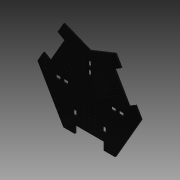
# Autodesk Inventor part: Bottom Plate
Saved by Autodesk Inventor 2015 (Build 190159000, 159)
## iProperties
Created: 2016-02-25
Part Number: Bottom Plate
Material: Polycarbonate, Clear
Document SubType Name: Modeling
Designer: James Yelland
Density: 1.2 g/cm^3
Appearance: Polycarbonate - Clear
Mass: 78.7459 g
Surface Area: 479.492 cm^2
Volume: 65.6216 cm^3
Author: James Yelland
Autodesk Inventor part; units mm, degrees
ref_plane "YZ Plane" through (0, 0, 0) normal (1, 0, 0) x (0, 1, 0)
ref_plane "XZ Plane" through (0, 0, 0) normal (0, 1, 0) x (-1, 0, 0)
ref_plane "XY Plane" through (0, 0, 0) normal (0, 0, 1) x (1, 0, 0)
sketch "Sketch1" plane through (0, 0, 0) normal (0, 1, 0) x (-1, 0, 0)
  line L0 (60.9555, 0.8544) -> (49.9555, 19.907)
  line L1 (-50.0445, 19.907) -> (-61.0445, 0.8544)
  line L2 (-28.0445, -153.2981) -> (-50.0445, -153.2981)
  line L3 (-50.0445, -153.2981) -> (-100.0445, -66.6956)
  line L4 (27.9555, -153.2981) -> (49.9555, -153.2981)
  line L5 (49.9555, -153.2981) -> (99.9555, -66.6956)
  line L6 (-100.0445, -66.6956) -> (-89.0445, -47.643)
  line L7 (88.9555, -47.643) -> (99.9555, -66.6956)
  line L8 (-0.0445, -0.093) -> (-50.0445, 19.907)
  line L9 (-0.0445, -0.093) -> (49.9555, 19.907)
  circle A0 centre (-66.9644, -113.992) radius 1.6
  circle A1 centre (-59.4644, -126.9824) radius 1.6
  circle A2 centre (59.3754, -126.9824) radius 1.6
  circle A3 centre (66.8754, -113.992) radius 1.6
  circle A4 centre (-49.2144, 11.3448) radius 1.6
  circle A5 centre (49.1254, 11.3448) radius 1.6
  circle A6 centre (-85.1445, -61.6956) radius 1.6
  circle A7 centre (-85.1445, -71.6956) radius 1.6
  circle A8 centre (85.0555, -61.6956) radius 1.6
  circle A9 centre (85.0555, -71.6956) radius 1.6
  circle A10 centre (-56.5116, -34.0943) radius 1.65
  circle A11 centre (-51.0123, -37.2693) radius 1.65
  circle A12 centre (-45.513, -40.4443) radius 1.65
  circle A13 centre (-40.0138, -43.6193) radius 1.65
  circle A14 centre (-34.5145, -46.7943) radius 1.65
  circle A15 centre (-29.0152, -49.9693) radius 1.65
  circle A16 centre (-23.516, -53.1443) radius 1.65
  circle A17 centre (-20.9056, -42.1229) radius 1.7
  circle A18 centre (-26.4048, -38.9479) radius 1.7
  circle A19 centre (-31.9041, -35.7729) radius 1.7
  circle A20 centre (-37.4034, -32.5979) radius 1.7
  circle A21 centre (-42.9026, -29.4229) radius 1.7
  circle A22 centre (-48.4019, -26.2479) radius 1.7
  circle A23 centre (-59.2519, -45.0407) radius 1.7
  circle A24 centre (-53.7526, -48.2157) radius 1.7
  circle A25 centre (-48.2534, -51.3907) radius 1.7
  circle A26 centre (-42.7541, -54.5657) radius 1.7
  circle A27 centre (-37.2548, -57.7407) radius 1.7
  circle A28 centre (-31.7556, -60.9157) radius 1.7
  line L10 (-62.0541, -30.8943) -> (-48.0541, -6.6456)
  line L11 (-48.0541, -6.6456) -> (-61.0445, 0.8544)
  line L12 (-62.0541, -30.8943) -> (-76.0541, -55.143)
  line L13 (-76.0541, -55.143) -> (-89.0445, -47.643)
  line L14 (-0.0445, -138.2981) -> (27.9555, -138.2981)
  line L15 (27.9555, -138.2981) -> (27.9555, -153.2981)
  line L16 (-0.0445, -138.2981) -> (-28.0445, -138.2981)
  line L17 (-28.0445, -138.2981) -> (-28.0445, -153.2981)
  line L18 (61.9651, -30.8943) -> (75.9651, -55.143)
  line L19 (75.9651, -55.143) -> (88.9555, -47.643)
  line L20 (61.9651, -30.8943) -> (47.9651, -6.6456)
  line L21 (47.9651, -6.6456) -> (60.9555, 0.8544)
  circle A29 centre (56.4226, -34.0943) radius 1.65
  circle A30 centre (50.9233, -37.2693) radius 1.65
  circle A31 centre (45.424, -40.4443) radius 1.65
  circle A32 centre (39.9248, -43.6193) radius 1.65
  circle A33 centre (34.4255, -46.7943) radius 1.65
  circle A34 centre (28.9263, -49.9693) radius 1.65
  circle A35 centre (23.427, -53.1443) radius 1.65
  circle A36 centre (31.6666, -60.9157) radius 1.7
  circle A37 centre (37.1658, -57.7407) radius 1.7
  circle A38 centre (42.6651, -54.5657) radius 1.7
  circle A39 centre (48.1644, -51.3907) radius 1.7
  circle A40 centre (53.6636, -48.2157) radius 1.7
  circle A41 centre (59.1629, -45.0407) radius 1.7
  circle A42 centre (48.3129, -26.2479) radius 1.7
  circle A43 centre (42.8136, -29.4229) radius 1.7
  circle A44 centre (37.3144, -32.5979) radius 1.7
  circle A45 centre (31.8151, -35.7729) radius 1.7
  circle A46 centre (26.3158, -38.9479) radius 1.7
  circle A47 centre (20.8166, -42.1229) radius 1.7
  circle A48 centre (-0.0445, -131.8981) radius 1.65
  circle A49 centre (-0.0445, -125.5481) radius 1.65
  circle A50 centre (-0.0445, -119.1981) radius 1.65
  circle A51 centre (-0.0445, -112.8481) radius 1.65
  circle A52 centre (-0.0445, -106.4981) radius 1.65
  circle A53 centre (-0.0445, -100.1481) radius 1.65
  circle A54 centre (-0.0445, -93.7981) radius 1.65
  circle A55 centre (-10.8945, -97.0481) radius 1.7
  circle A56 centre (-10.8945, -103.3981) radius 1.7
  circle A57 centre (-10.8945, -109.7481) radius 1.7
  circle A58 centre (-10.8945, -116.0981) radius 1.7
  circle A59 centre (-10.8945, -122.4481) radius 1.7
  circle A60 centre (-10.8945, -128.7981) radius 1.7
  circle A61 centre (10.8055, -128.7981) radius 1.7
  circle A62 centre (10.8055, -122.4481) radius 1.7
  circle A63 centre (10.8055, -116.0981) radius 1.7
  circle A64 centre (10.8055, -109.7481) radius 1.7
  circle A65 centre (10.8055, -103.3981) radius 1.7
  circle A66 centre (10.8055, -97.0481) radius 1.7
  line L22 (-62.0541, -30.8943) -> (-68.3041, -41.7196)
  line L23 (-66.0445, -71.6956) -> (-66.0445, -78.6956)
  line L24 (-66.0445, -78.6956) -> (-56.0445, -78.6956)
  line L25 (-56.0445, -78.6956) -> (-56.0445, -71.6956)
  line L26 (-56.0445, -71.6956) -> (-66.0445, -71.6956)
  line L27 (-51.0445, -71.6956) -> (-51.0445, -78.6956)
  line L28 (-51.0445, -78.6956) -> (-41.0445, -78.6956)
  line L29 (-41.0445, -78.6956) -> (-41.0445, -71.6956)
  line L30 (-41.0445, -71.6956) -> (-51.0445, -71.6956)
  line L31 (65.9555, -71.6956) -> (65.9555, -78.6956)
  line L32 (65.9555, -78.6956) -> (55.9555, -78.6956)
  line L33 (55.9555, -78.6956) -> (55.9555, -71.6956)
  line L34 (55.9555, -71.6956) -> (65.9555, -71.6956)
  line L35 (50.9555, -71.6956) -> (50.9555, -78.6956)
  line L36 (50.9555, -78.6956) -> (40.9555, -78.6956)
  line L37 (40.9555, -78.6956) -> (40.9555, -71.6956)
  line L38 (40.9555, -71.6956) -> (50.9555, -71.6956)
  line L39 (-0.0445, -17.093) -> (3.4555, -17.093)
  line L40 (3.4555, -17.093) -> (3.4555, -27.093)
  line L41 (3.4555, -27.093) -> (-3.5445, -27.093)
  line L42 (-3.5445, -27.093) -> (-3.5445, -17.093)
  line L43 (-3.5445, -17.093) -> (-0.0445, -17.093)
  line L44 (-0.0445, -32.093) -> (3.4555, -32.093)
  line L45 (3.4555, -32.093) -> (3.4555, -42.093)
  line L46 (3.4555, -42.093) -> (-3.5445, -42.093)
  line L47 (-3.5445, -42.093) -> (-3.5445, -32.093)
  line L48 (-3.5445, -32.093) -> (-0.0445, -32.093)
  line L49 (-25.0445, -123.2981) -> (-25.0445, -113.2981)
  line L50 (-25.0445, -113.2981) -> (-32.0445, -113.2981)
  line L51 (-32.0445, -113.2981) -> (-32.0445, -123.2981)
  line L52 (-32.0445, -123.2981) -> (-25.0445, -123.2981)
  line L53 (24.9555, -123.2981) -> (24.9555, -113.2981)
  line L54 (24.9555, -113.2981) -> (31.9555, -113.2981)
  line L55 (31.9555, -113.2981) -> (31.9555, -123.2981)
  line L56 (31.9555, -123.2981) -> (24.9555, -123.2981)
  circle A67 centre (-37.0445, -113.2981) radius 1.6
  circle A68 centre (-20.0445, -123.2981) radius 1.6
  circle A69 centre (36.9555, -113.2981) radius 1.6
  circle A70 centre (19.9555, -123.2981) radius 1.6
  circle A71 centre (-12.0445, -56.7981) radius 1.6
  circle A72 centre (11.9555, -80.7981) radius 1.6
  circle A73 centre (-64.0445, -66.6956) radius 1.6
  circle A74 centre (-43.0445, -83.6956) radius 1.6
  circle A75 centre (63.9555, -66.6956) radius 1.6
  circle A76 centre (42.9555, -83.6956) radius 1.6
  circle A77 centre (-8.5445, -19.093) radius 1.6
  circle A78 centre (8.4555, -40.093) radius 1.6
  constraints: 114 end point, 79 centre point, 7 point on line
extrude "Extrusion2" add sketch "Sketch1" along normal blind 3
body "Solid2"
